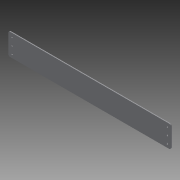
# Autodesk Inventor part: Metal E-board
Saved by Autodesk Inventor 2015 (Build 190159000, 159)
## iProperties
Created: 2015-02-08
Part Number: Metal E-board
Material: Generic
Document SubType Name: Modeling
Designer: whitaus15
Density: 1 g/cm^3
Appearance: Default
Author: whitaus15
Autodesk Inventor part; units mm, degrees
ref_plane "YZ Plane" through (0, 0, 0) normal (1, 0, 0) x (0, 1, 0)
ref_plane "XZ Plane" through (0, 0, 0) normal (0, 1, 0) x (-1, 0, 0)
ref_plane "XY Plane" through (0, 0, 0) normal (0, 0, 1) x (1, 0, 0)
sketch "Sketch1" plane through (0, 0, 0) normal (0, 0, 1) x (1, 0, 0)
  line L0 (0, 0) -> (566.42, 0)
  line L1 (566.42, 0) -> (566.42, 330.2)
  line L2 (566.42, 330.2) -> (0, 330.2)
  line L3 (0, 330.2) -> (0, 0)
  dimension "d0" = 330.2
  dimension "d1" = 566.42
  constraints: 8 end point, 2 parallel, 1 horizontal, 1 perpendicular
  measures "d0" distance of L2.end L0.start
  measures "d1" distance of L0.start L0.end
extrude "Extrusion1" add sketch "Sketch1" along normal blind 3.175
sketch "Sketch3" plane through (0, 0, 3.175) normal (0, 0, 1) x (1, 0, 0)
  line L0 (566.42, 330.2) -> (553.72, 330.2)
  line L1 (553.72, 330.2) -> (553.72, 317.5)
  line L2 (553.72, 317.5) -> (566.42, 317.5)
  line L3 (566.42, 317.5) -> (566.42, 330.2)
  circle A0 centre (553.72, 317.5) radius 3.175
  point P0 (0, 0)
  dimension "d4" = 12.7
  dimension "d5" = 12.7
  dimension "d6" = 6.35
  constraints: 8 end point, 2 parallel, 1 centre point, 1 coincident, 1 horizontal, 1 perpendicular
  measures "d4" distance of L0.end L1.end
  measures "d5" distance of L1.end L2.end
  measures "d6" diameter of A0
extrude "Extrusion2" cut sketch "Sketch3" against normal through all contours A0 L2 L1 | L1 L2 A0
pattern_linear "Rectangular Pattern1" count 5 spacing 76.2 along (0, -1, 0) count 2 spacing 541.02 along (-1, 0, 0) of "Extrusion2"
sketch "Sketch4" plane through (0, 0, 3.175) normal (0, 0, 1) x (1, 0, 0)
  line L0 (566.42, 330.2) -> (553.72, 330.2)
  line L1 (553.72, 330.2) -> (553.72, 266.7)
  line L2 (553.72, 266.7) -> (566.42, 266.7)
  line L3 (566.42, 266.7) -> (566.42, 330.2)
  circle A0 centre (553.72, 266.7) radius 6.35
  point P0 (0, 0)
  dimension "d15" = 12.7
  dimension "d16" = 63.5
  dimension "d17" = 12.7
  constraints: 8 end point, 2 parallel, 1 centre point, 1 coincident, 1 horizontal, 1 perpendicular
  measures "d15" distance of L1.end L2.end
  measures "d16" distance of L0.end L1.end
  measures "d17" diameter of A0
extrude "Extrusion3" cut sketch "Sketch4" against normal through all contours A0 L2 L1 | L1 L2 A0
pattern_linear "Rectangular Pattern2" count 2 spacing 541.02 along (-1, 0, 0) of "Extrusion3"
sketch "Sketch6" plane through (0, 0, 3.175) normal (0, 0, 1) x (1, 0, 0)
  line L0 (566.42, 0) -> (566.42, 330.2) projected
  line L1 (0, 0) -> (566.42, 0)
  line L2 (566.42, 0) -> (566.42, 76.2)
  line L3 (566.42, 76.2) -> (0, 76.2)
  line L4 (0, 76.2) -> (0, 0)
  line L5 (0, 76.2) -> (566.42, 76.2)
  line L6 (566.42, 76.2) -> (566.42, 330.2)
  line L7 (566.42, 330.2) -> (0, 330.2)
  line L8 (0, 330.2) -> (0, 76.2)
  dimension "d23" = 76.2
  constraints: 16 end point, 4 parallel, 2 horizontal, 2 perpendicular, 1 point on line
  measures "d23" distance between parallel lines of L1 L3
extrude "Extrusion4" cut sketch "Sketch6" against normal through all contours L3 L8 L7 L0
sketch "Sketch7" plane through (0, 0, 3.175) normal (0, 0, 1) x (1, 0, 0)
  line L0 (0, 0) -> (566.42, 0) projected
  line L1 (283.21, 0) -> (283.21, 76.2)
  line L2 (566.42, 76.2) -> (0, 76.2) projected
  line L3 (283.21, 76.2) -> (389.89, 76.2)
  line L4 (389.89, 76.2) -> (176.53, 76.2)
  line L5 (176.53, 76.2) -> (176.53, 63.5)
  line L6 (389.89, 76.2) -> (389.89, 63.5)
  circle A0 centre (176.53, 63.5) radius 3.175
  circle A1 centre (389.89, 63.5) radius 3.175
  line L7 (176.53, 63.5) -> (176.53, 18.796)
  circle A2 centre (176.53, 18.796) radius 3.175
  circle A3 centre (389.89, 18.796) radius 3.175
  dimension "d26" = 106.68
  dimension "d27" = 213.36
  dimension "d28" = 12.7
  dimension "d29" = 12.7
  dimension "d30" = 6.35
  dimension "d31" = 6.35
  dimension "d34" = 44.704
  dimension "d35" = 6.35
  constraints: 12 end point, 4 centre point, 3 coincident, 2 midpoint, 2 point on line, 1 parallel, 1 perpendicular, 1 symmetric about line, 1 vertical, 1 other
  measures "d26" distance of L1.end L3.end
  measures "d27" distance of L3.end L4.end
  measures "d28" distance of L4.end L5.end
  measures "d29" distance of L3.end L6.end
  measures "d30" diameter of A0
  measures "d31" diameter of A1
  measures "d34" distance of L7.start L7.end
  measures "d35" diameter of A2
extrude "Extrusion6" cut sketch "Sketch7" against normal through all
sketch "Sketch9" plane through (0, 0, 3.175) normal (0, 0, 1) x (1, 0, 0)
  circle A0 centre (12.7, 12.7) radius 3.175 projected
  line L0 (12.7, 12.7) -> (12.7, 38.1)
  line L1 (12.7, 38.1) -> (12.7, 63.5)
  circle A1 centre (12.7, 63.5) radius 3.175
  circle A2 centre (12.7, 38.1) radius 3.175
  line L2 (0, 0) -> (566.42, 0) projected
  line L3 (283.21, 0) -> (283.21, 76.2)
  line L4 (0, 76.2) -> (566.42, 76.2) projected
  circle A3 centre (553.72, 12.7) radius 3.175
  circle A4 centre (553.72, 63.5) radius 3.175
  circle A5 centre (553.72, 38.1) radius 3.175
  dimension "d45" = 25.4
  dimension "d46" = 25.4
  dimension "d47" = 6.35
  dimension "d48" = 6.35
  constraints: 6 end point, 5 centre point, 3 symmetric about line, 2 coincident, 2 midpoint, 1 point on line, 1 vertical, 3 other
  measures "d45" distance of L0.start L0.end
  measures "d46" distance of L0.end L1.end
  measures "d47" diameter of A1
  measures "d48" diameter of A2
extrude "Extrusion8" cut sketch "Sketch9" against normal through all contours A1 | A2 L1 L0 | L0 L1 A2 | A4 | A5
sketch "Sketch12" plane through (0, 0, 3.175) normal (0, 0, 1) x (1, 0, 0)
  line L0 (566.42, 76.2) -> (0, 76.2) projected
  line L1 (283.21, 76.2) -> (283.21, 0)
  line L2 (50.8, 57.15) -> (109.4994, 57.15)
  line L3 (80.1497, 57.15) -> (80.1497, 76.2)
  line L4 (0, 76.2) -> (0, 0) projected
  circle A0 centre (50.8, 57.15) radius 2.5019
  circle A1 centre (109.4994, 57.15) radius 2.5019
  circle A2 centre (515.62, 57.15) radius 2.5019
  circle A3 centre (456.9206, 57.15) radius 2.5019
  dimension "d85" = 19.05
  dimension "d86" = 58.6994
  dimension "d87" = 50.8
  dimension "d88" = 5.0038
  dimension "d89" = 5.0038
  constraints: 6 end point, 4 centre point, 4 coincident, 4 symmetric about line, 2 midpoint, 1 horizontal, 1 perpendicular, 1 point on line, 1 vertical, 2 other
  measures "d85" distance of L3.start L3.end
  measures "d86" distance of L2.start L2.end
  measures "d87" distance from line of L4 L2.start
  measures "d88" diameter of A0
  measures "d89" diameter of A1
extrude "Extrusion11" cut sketch "Sketch12" against normal through all
fillet "Fillet1" radius 6.35 4 edges at (0, 76.2, 1.5875) (0, 0, 1.5875) (566.42, 76.2, 1.5875) (566.42, 0, 1.5875)
sketch "Sketch13" plane through (0, 0, 3.175) normal (0, 0, 1) x (1, 0, 0)
  line L0 (33.566, 68.6086) -> (529.2252, 68.6086)
  line L1 (529.2252, 68.6086) -> (529.2252, 9.2074)
  line L2 (529.2252, 9.2074) -> (33.566, 9.2074)
  line L3 (33.566, 9.2074) -> (33.566, 68.6086)
  point P0 (0, 0)
  constraints: 8 end point, 2 parallel, 1 horizontal, 1 perpendicular
extrude "Extrusion12" add sketch "Sketch13" against normal blind 3.175
body "Solid1"
